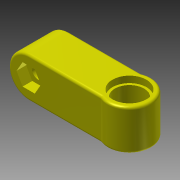
# Autodesk Inventor part: hub center
Saved by Autodesk Inventor 2013 (Build 170138000, 138)
## iProperties
Created: 2013-07-14
Part Number: hub center
Material: Generic
Document SubType Name: Modeling
Designer: employee
Density: 1 g/cm^3
Author: employee
Autodesk Inventor part; units mm, degrees
ref_plane "YZ Plane" through (0, 0, 0) normal (1, 0, 0) x (0, 1, 0)
ref_plane "XZ Plane" through (0, 0, 0) normal (0, 1, 0) x (-1, 0, 0)
ref_plane "XY Plane" through (0, 0, 0) normal (0, 0, 1) x (1, 0, 0)
sketch "Sketch1" plane through (0, 0, 0) normal (0, 0, 1) x (1, 0, 0)
  line L0 (0, 0) -> (0, 12.5)
  line L1 (0, 12.5) -> (50, 12.5)
  arc A0 (50, -12.5) -> (50, 12.5) centre (50, 0) ccw
  line L2 (50, -12.5) -> (0, -12.5)
  line L3 (0, -12.5) -> (0, 0)
  dimension "d0" = 12.5
  dimension "d2" = 50
  constraints: 8 end point, 2 equal length, 2 point on circle, 2 tangent, 1 centre point, 1 collinear, 1 perpendicular, 1 vertical
  measures "d0" radius of A0
  measures "d2" distance of L0.end L1.end
extrude "Extrusion1" add sketch "Sketch1" along normal blind 25
sketch "Sketch2" plane through (0, -12.5, 0) normal (0, -1, 0) x (1, 0, 0)
  line L0 (0, 0) -> (0, 25) projected
  circle A0 centre (0, 12.5) radius 12.5
  constraints: 1 midpoint, 1 vertical alignment, 2 other
extrude "Extrusion2" add sketch "Sketch2" against normal up to surface (25 mm away)
sketch "Sketch3" plane through (50, -12.5, 0) normal (0, -1, 0) x (1, 0, 0)
  arc A0 (-50, 25) -> (-50, 0) centre (-50, 12.5) ccw projected
  circle A1 centre (-50, 12.5) radius 4.05
  dimension "d7" = 8.1
  constraints: 1 centre point, 1 coincident
  measures "d7" diameter of A1
extrude "Extrusion3" cut sketch "Sketch3" against normal through all
sketch "Sketch4" plane through (0, 0, 25) normal (0, 0, 1) x (1, 0, 0)
  arc A0 (50, -12.5) -> (50, 12.5) centre (50, 0) ccw projected
  circle A1 centre (50, 0) radius 9.05
  point P0 (0, 0)
  dimension "d11" = 18.1
  constraints: 1 centre point, 1 coincident
  measures "d11" diameter of A1
extrude "Extrusion4" cut sketch "Sketch4" against normal through all
sketch "Sketch16" plane through (50, -12.5, 0) normal (0, -1, 0) x (1, 0, 0)
  circle A0 centre (-50, 12.5) radius 4.05 projected
  arc A1 (-50, 25) -> (-50, 0) centre (-50, 12.5) ccw projected
  line L0 (-57.5633, 12.5) -> (-53.7816, 19.05)
  line L1 (-53.7816, 19.05) -> (-46.2184, 19.05)
  line L2 (-46.2184, 19.05) -> (-42.4367, 12.5)
  line L3 (-42.4367, 12.5) -> (-46.2184, 5.95)
  line L4 (-46.2184, 5.95) -> (-53.7816, 5.95)
  line L5 (-53.7816, 5.95) -> (-57.5633, 12.5)
  dimension "d74" = 13.1
  constraints: 12 end point, 1 coincident, 1 horizontal, 13 other
  measures "d74" distance between parallel lines of L1 L4
extrude "Extrusion14" cut sketch "Sketch16" against normal blind 6
sketch "Sketch17" plane through (0, 0, 25) normal (0, 0, 1) x (1, 0, 0)
  circle A0 centre (50, 0) radius 9.05 projected
  arc A1 (50, -12.5) -> (50, 12.5) centre (50, 0) ccw projected
  circle A2 centre (50, 0) radius 10.55
  point P0 (0, 0)
  dimension "d78" = 21.1
  constraints: 1 centre point, 1 coincident
  measures "d78" diameter of A2
extrude "Extrusion15" cut sketch "Sketch17" against normal blind 4
sketch "Sketch19" plane through (0, 0, 0) normal (0, 0, -1) x (-1, 0, 0)
  circle A0 centre (-50, 0) radius 9.05 projected
  circle A1 centre (-50, 0) radius 10.55 projected
  point P0 (0, 0)
extrude "Extrusion16" cut sketch "Sketch19" against normal blind 4
chamfer "Chamfer2" distance 1.5 angle 45 1 edges at (40.95, 0, 4)
sketch "Sketch20" plane through (0, 0, 25) normal (0, 0, 1) x (1, 0, 0)
  circle A0 centre (50, 0) radius 10.55 projected
  arc A1 (50, -12.5) -> (50, 12.5) centre (50, 0) ccw projected
  circle A2 centre (50, 0) radius 13.55
  point P0 (0, 0)
  dimension "d87" = 3
  constraints: 1 centre point, 1 coincident
  measures "d87" radial gap between concentric circles of A2 A0
extrude "Extrusion17" add sketch "Sketch20" against normal up to surface (25 mm away)
fillet "Fillet1" radius 1.5 10 edges at (22.385, 12.5, 25) (22.385, -12.5, 25) (63.55, 0, 25) (-12.5, 12.5, 12.5) (22.385, 12.5, 0) (-12.5, -12.5, 12.5) (22.385, -12.5, 0) (44.77, 12.5, 12.5) (44.77, -12.5, 12.5) (63.55, 0, 0)
body "Solid1"
